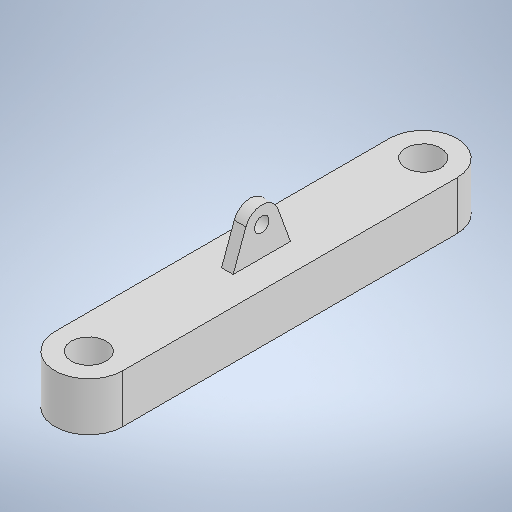
# Autodesk Inventor part: Gripper_arms
Saved by Autodesk Inventor 2025.2 (Build 292293000, 293)
## iProperties
Created: 2025-01-12
Part Number: Gripper_arms
Material: Generic
Document SubType Name: Modeling
Designer: caomi
Density: 1 g/cm^3
Appearance: Default
Author: caomi
Autodesk Inventor part; units mm, degrees
ref_plane "YZ Plane" through (0, 0, 0) normal (1, 0, 0) x (0, 1, 0)
ref_plane "XZ Plane" through (0, 0, 0) normal (0, 1, 0) x (-1, 0, 0)
ref_plane "XY Plane" through (0, 0, 0) normal (0, 0, 1) x (1, 0, 0)
sketch "Sketch1" plane through (0, 0, 0) normal (0, 1, 0) x (-1, 0, 0)
  line L0 (-7, 41.5) -> (7, 41.5)
  line L1 (7, 41.5) -> (7, -41.5)
  line L2 (7, -41.5) -> (-7, -41.5)
  line L3 (-7, -41.5) -> (-7, 41.5)
  line L4 (-7, 41.5) -> (7, -41.5) construction
  line L5 (7, 41.5) -> (-7, -41.5) construction
  circle A0 centre (0, 34.5) radius 3.6
  circle A1 centre (0, -34.5) radius 3.6
  line L6 (13.7936, 0) -> (-15.5073, 0) construction
  point P0 (0, 0)
  dimension "d0" = 7.2
  dimension "d1" = 69
  dimension "d2" = 83
  dimension "d3" = 14
  constraints: 14 end point, 2 centre point, 2 horizontal, 2 midpoint, 2 parallel, 2 vertical alignment, 1 perpendicular, 1 point on line, 1 other
  measures "d0" diameter of A0
  measures "d1" distance of A0.centre A1.centre
  measures "d2" distance of L0.end L1.end
  measures "d3" distance of L0.start L0.end
extrude "Extrusion1" add sketch "Sketch1" along normal mid plane 10
sketch "Sketch2" plane through (0, 0, 0) normal (1, 0, 0) x (0, 1, 0)
  circle A0 centre (11, 0) radius 3.5
  line L0 (12.1971, -3.2889) -> (5, -5.9084)
  line L1 (5, -41.5) -> (5, 41.5) projected
  line L2 (12.1971, 3.2889) -> (5, 5.9084)
  line L3 (11, 0) -> (-7.9221, 0) construction
  circle A1 centre (11, 0) radius 1.5
  point P0 (0, 0)
  point P1 (16.3025, 1.2439)
  point P2 (5, 7.6173)
  point P3 (5, -5.09)
  point P4 (5, 0)
  dimension "d6" = 7
  dimension "d11" = 20
  dimension "d12" = 6
  dimension "d13" = 3
  constraints: 6 end point, 2 centre point, 2 point on circle, 2 point on line, 1 horizontal, 1 horizontal alignment, 1 midpoint, 1 tangent, 1 other
  measures "d6" diameter of A0
  measures "d11" angle of L3 L2
  measures "d12" distance of point (5, 0) L3.start
  measures "d13" diameter of A1
extrude "Extrusion2" add sketch "Sketch2" along normal mid plane 2.4
fillet "Fillet1" radius 7 4 edges at (-7, 0, 41.5) (7, 0, 41.5) (-7, 0, -41.5) (7, 0, -41.5)
equation "\"d10\" = 0.5 * d3"
body "Solid1"
